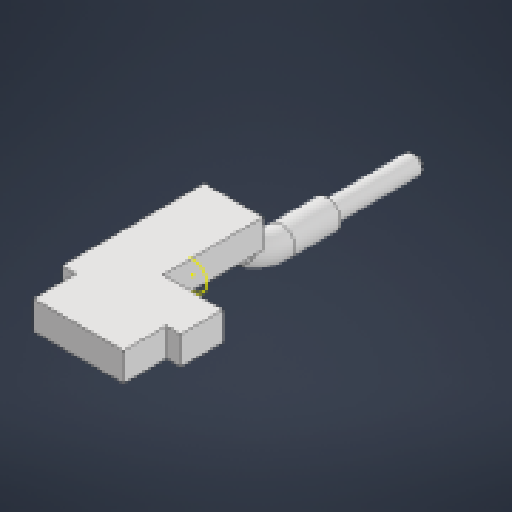
# Autodesk Inventor part: 轴系按钮2
Saved by Autodesk Inventor 2025 (Build 290162000, 162)
## iProperties
Created: 2026-04-16
Part Number: 轴系按钮2
Material: 常规
Document SubType Name: Modeling
Designer: XH
Density: 1 g/cm^3
Appearance: 默认
Author: XH
Autodesk Inventor part; units mm, degrees
ref_plane "YZ Plane" through (0, 0, 0) normal (1, 0, 0) x (0, 1, 0)
ref_plane "XZ Plane" through (0, 0, 0) normal (0, 1, 0) x (-1, 0, 0)
ref_plane "XY Plane" through (0, 0, 0) normal (0, 0, 1) x (1, 0, 0)
sketch "草图1" plane through (0, 0, 0) normal (0, 0, 1) x (1, 0, 0)
  line L0 (4.75, -1.5) -> (-4.75, -1.5)
  line L1 (-4.75, -1.5) -> (-4.75, 1.5)
  line L2 (-4.75, 1.5) -> (4.75, 1.5)
  line L3 (4.75, 1.5) -> (4.75, -1.5)
  line L4 (4.75, -1.5) -> (-4.75, 1.5) construction
  line L5 (-4.75, -1.5) -> (4.75, 1.5) construction
  circle A0 centre (0, 0) radius 1
  dimension "d0" = 3
  dimension "d1" = 2
  dimension "d2" = 9.5
  constraints: 12 end point, 2 midpoint, 2 parallel, 1 centre point, 1 coincident, 1 horizontal, 1 perpendicular
  measures "d0" distance of L2.end L0.start
  measures "d1" diameter of A0
  measures "d2" distance of L1.end L2.end
extrude "拉伸1" add sketch "草图1" along normal blind 3
sketch "草图2" plane through (0, 0, 3) normal (0, 0, 1) x (1, 0, 0)
  line L0 (4.75, 1.5) -> (-4.75, 1.5) projected
  line L1 (-4.75, 1.5) -> (-4.75, -1.5) projected
  line L2 (-4.75, -1.5) -> (4.75, -1.5) projected
  line L3 (4.75, -1.5) -> (4.75, 1.5) projected
  circle A0 centre (0, 0) radius 1 projected
extrude "拉伸2" add sketch "草图2" along normal blind 10 contours L3 L2 L1 L0 | A0
sketch "草图3" plane through (-4.75, 1.5, 0) normal (0, 1, 0) x (1, 0, 0)
  line L0 (-1.5, 0) -> (11, 0)
  line L1 (11, 0) -> (11, -7)
  line L2 (11, -7) -> (-1.5, -7)
  line L3 (-1.5, -7) -> (-1.5, 0)
  line L4 (9.5, 0) -> (9.5, -13) projected
  line L5 (0, 0) -> (0, -13) projected
  line L6 (9.5, 0) -> (0, 0) projected
  point P0 (4.75, 0)
  point P1 (-1.5, -3.5)
  point P2 (9.5, -7)
  point P3 (0, -7)
  dimension "d8" = 1.5
  dimension "d9" = 1.5
  dimension "d15" = 7
  constraints: 8 end point, 2 parallel, 1 collinear, 1 horizontal, 1 midpoint, 1 perpendicular
  measures "d8" distance between parallel lines of L4 L1
  measures "d9" distance from line of L5 point (-1.5, -3.5)
  measures "d15" distance between parallel lines of L2 L0
extrude "拉伸3" add sketch "草图3" against normal blind 3
move faces "移动1" translate (0, 0, 2) faces at (1.5833, 0.5, 13)
sketch "草图4" plane through (0, 0, 0) normal (0, 0, -1) x (-1, 0, 0)
  circle A0 centre (0, 0) radius 1.5
  dimension "d16" = 3
  constraints: 1 centre point, 1 coincident
  measures "d16" diameter of A0
extrude "拉伸4" add sketch "草图4" along normal blind 0.5
ref_plane "工作平面1" through (11.9199, 26.93, -22.8525) normal (0, 0, 1) x (-1, 0, 0)
sketch "草图5" plane through (11.9199, 26.93, -22.8525) normal (0, 0, 1) x (-1, 0, 0)
  circle A0 centre (13.6237, 30.1067) radius 1.5
  circle A1 centre (13.716, 24.2534) radius 1.5
  circle A2 centre (13.6237, 30.1067) radius 1.5
  point P0 (11.9199, 26.93)
  dimension "d19" = 3
  constraints: 3 centre point, 1 coincident, 3 other
  measures "d19" diameter of A0
sketch "草图7" plane through (0, 0, -0.5) normal (0, 0, -1) x (-1, 0, 0)
  circle A0 centre (0, 0) radius 1.5 projected
ref_plane "工作平面2" through (11.9199, 26.93, -12.8525) normal (0, 0, 1) x (-1, 0, 0)
sketch "草图8" plane through (11.9199, 26.93, -12.8525) normal (0, 0, 1) x (-1, 0, 0)
  circle A0 centre (12.3625, 23.27) radius 1.5
  point P0 (11.9199, 26.93)
  constraints: 1 centre point
sketch "草图9" plane through (0, 0, 0) normal (1, 0, 0) x (0, 1, 0)
  line L0 (-4.6767, -22.8525) -> (-1.6767, -22.8525) projected
  line L1 (-3.1767, -22.8525) -> (-3.1767, -11.5324)
  arc A0 (-1.651, -7.3854) -> (-3.1767, -11.5324) centre (3.2225, -11.5324) ccw
  arc A1 (-1.651, -7.3854) -> (0.0125, -4.1729) centre (-6.1762, -3.0051) ccw
  point P0 (-3.6148, -22.5313)
  point P1 (-2.7659, -4.1729)
  constraints: 4 point on circle, 2 centre point, 2 end point, 1 midpoint, 1 tangent, 1 vertical
sweep "扫掠1" add profiles "草图5" path "草图9" path curves L1 A0 A1 contours A0
loft "放样1" add section 1 edges at (1.5, 0, -0.5) section 2 edges at (-0.2038, 0.0125, -4.1729)
sketch "草图15" plane through (0, 0, 0) normal (0, 0, -1) x (-1, 0, 0)
  line L0 (-6.25, 1.5) -> (0, 1.5) projected
  line L1 (4.75, -1.5) -> (6.25, -1.5) projected
  line L2 (-6.25, 1.5) -> (6.25, 1.5)
  line L3 (6.25, 1.5) -> (6.25, -1.5)
  line L4 (6.25, -1.5) -> (-6.25, -1.5)
  line L5 (-6.25, -1.5) -> (-6.25, 1.5)
  point P0 (0, 0)
  point P1 (0, 1.5)
  constraints: 8 end point, 2 parallel, 1 horizontal, 1 perpendicular
extrude "拉伸9" add sketch "草图15" along normal blind 8
sketch "草图16" plane through (4.75, 1.5, 7) normal (0, 1, 0) x (1, 0, 0)
  line L0 (1.5, 15) -> (-11, 15) projected
  line L1 (1.5, 15) -> (-4.829, 15)
  line L2 (-4.829, 15) -> (-4.829, 4.4703)
  line L3 (-4.829, 4.4703) -> (1.5, 4.4703)
  line L4 (1.5, 4.4703) -> (1.5, 15)
  point P0 (-4.75, 7)
  constraints: 8 end point, 2 parallel, 1 horizontal, 1 perpendicular, 1 point on line
extrude "拉伸10" cut sketch "草图16" against normal blind 6.75
sketch "草图17" plane through (-1.7038, -3.1767, -22.8525) normal (0, 0, -1) x (-1, 0, 0)
  circle A0 centre (0, 0) radius 1.5 projected
  circle A1 centre (0, 0) radius 1
  point P0 (-1.7038, 3.1767)
  dimension "d46" = 2
  constraints: 1 centre point, 1 coincident
  measures "d46" diameter of A1
ref_plane "工作平面3" through (0.201, 1.0367, -16.3525) normal (0, 0, -1) x (0, 1, 0)
extrude "拉伸11" cut sketch "草图17" against normal up to surface (6.5 mm away)
sketch "草图18" plane through (-1.7038, -3.1767, -16.3525) normal (0, 0, -1) x (-1, 0, 0)
  circle A0 centre (0, 0) radius 1 projected
  point P0 (-1.7038, 3.1767)
extrude "拉伸12" add sketch "草图18" along normal blind 9.5
chamfer "倒角2" distance 0.5 angle 45 1 edges at (-0.7038, -3.1767, -25.8525)
offset faces "大小2" outward -3.5 faces at (1.5833, -0.5, 15)
offset faces "大小3" outward 1 faces at (1.5833, -0.5, 11.5)
